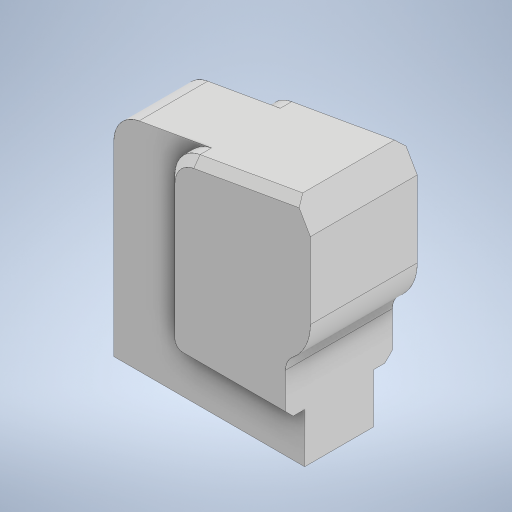
# Autodesk Inventor part: Idler Block Left
Saved by Autodesk Inventor 2024 (Build 280153000, 153)
## iProperties
Created: 2024-08-12
Part Number: Idler Block Left
Material: Generic
Document SubType Name: Modeling
Designer: Ishaan
Density: 1 g/cm^3
Appearance: Default
Author: Ishaan
Autodesk Inventor part; units mm, degrees
ref_plane "YZ Plane" through (0, 0, 0) normal (1, 0, 0) x (0, 1, 0)
ref_plane "XZ Plane" through (0, 0, 0) normal (0, 1, 0) x (-1, 0, 0)
ref_plane "XY Plane" through (0, 0, 0) normal (0, 0, 1) x (1, 0, 0)
sketch "Sketch1" plane through (0, 0, 0) normal (0, 0, 1) x (1, 0, 0)
  circle A0 centre (0, 0) radius 12.5
  circle A1 centre (0, 0) radius 25
  line L0 (-25, 0) -> (6, 0)
  line L1 (6, 0) -> (6, -25)
  line L2 (6, -25) -> (-25, -25)
  line L3 (-25, -25) -> (-25, 0)
  line L4 (12.5, 0) -> (12.5, 19.9562)
  line L5 (12.5, 19.9562) -> (8.5, 26.8844)
  line L6 (-4.3412, 24.6202) -> (8.5, 26.8844)
  line L7 (-25, 0) -> (-25, 20.9775)
  line L8 (-25, 20.9775) -> (-4.3412, 24.6202)
  line L9 (-20, -38) -> (0, -38) construction
  point P0 (6, -10.9659)
  point P1 (0, -25)
  point P2 (6, -24.2693)
  point P3 (-12.5, 0)
  dimension "d0" = 25
  dimension "d1" = 50
  dimension "d2" = 6
  dimension "d7" = 150
  dimension "d8" = 4
  dimension "d9" = 110
  dimension "d13" = 38
  constraints: 20 end point, 4 tangent, 2 coincident, 2 horizontal, 2 parallel, 2 point on circle, 2 vertical, 1 centre point, 1 collinear, 1 perpendicular, 1 point on line, 3 other
  measures "d1" diameter of A1
  measures "d2" distance from line of point (0, 0) L1
  measures "d7" angle of L4 L5
  measures "d8" distance from line of L4 L5.end
  measures "d9" angle of L5 L6
  measures "d13" distance from line of point (0, 0) L9
extrude "Extrusion1" add sketch "Sketch1" along normal mid plane 28 contours A0 L1 L0 | A0 L0 A1 L5 L4 | L0 L1 A0 | A0 L1 A1 L0 | L7 L8 A1 | A1 L2 L3 | L1 L2 A1 | A1 L6 L5
fillet "Fillet1" radius 5 1 edges at (6, -10.9659, 0)
sketch "Sketch2" plane through (0, 0, 0) normal (0, 0, 1) x (1, 0, 0)
  line L0 (8.5, 26.8844) -> (12.5, 19.9562) projected
  line L1 (12.5, 19.9562) -> (12.5, 0) projected
  arc A0 (7.8571, -9.7219) -> (12.5, 0) centre (0, 0) ccw projected
  arc A1 (7.8571, -9.7219) -> (6, -13.6107) centre (11, -13.6107) ccw projected
  line L2 (6, -13.6107) -> (6, -25) projected
  line L3 (6, -25) -> (-25, -25) projected
  line L4 (-25, -25) -> (-25, 20.9775) projected
  line L5 (-25, 20.9775) -> (8.5, 26.8844) projected
  line L6 (-25, 20.9775) -> (-44, 17.6273)
  line L7 (-44, 17.6273) -> (-44, -25)
  line L8 (-44, -25) -> (-25, -25)
  line L9 (8.5, 26.8844) -> (-25, 20.9775) projected
  line L10 (-44, -25) -> (6, -25)
  line L11 (6, -25) -> (6, -38)
  line L12 (6, -38) -> (-44, -38)
  line L13 (-44, -38) -> (-44, -25)
  line L14 (6, -25) -> (6, -13.6107) projected
  dimension "d14" = 38
  dimension "d21" = 50
  constraints: 14 end point, 2 collinear, 2 parallel, 2 perpendicular, 1 horizontal, 1 vertical
  measures "d14" distance from line of L12 point (0, 0)
  measures "d21" distance of L11.end L12.end
extrude "Extrusion2" add sketch "Sketch2" along normal mid plane 18 contours L4 L8 L7 L6 | L3 L11 L12 L13 L8
fillet "Fillet4" radius 8 3 edges at (-25, 20.9775, -11.5) (-25, 20.9775, 11.5) (-44, 17.6273, 0)
fillet "Fillet3" radius 4 2 edges at (-25, -25, 11.5) (-25, -25, -11.5)
chamfer "Chamfer1" distance 2 angle 45 10 edges at (-4.9446, 24.5138, -14) (-23.1284, 19.407, -14) (-25, -3.3677, -14) (-23.8284, -23.8284, -14) (-7.5, -25, -14) (-4.9446, 24.5138, 14) (-23.1284, 19.407, 14) (-25, -3.3677, 14) (-23.8284, -23.8284, 14) (-7.5, -25, 14)
body "Solid1"
